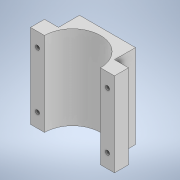
# Autodesk Inventor part: boltSideForclampForMeadeTripodLeg
Saved by Autodesk Inventor 2021.2 (Build 252289000, 289)
## iProperties
Created: 2021-02-07
Part Number: boltSideForclampForMeadeTripodLeg
Material: Generic
Document SubType Name: Modeling
Designer: robst
Density: 1 g/cm^3
Appearance: Default
Author: robst
Autodesk Inventor part; units mm, degrees
ref_plane "YZ Plane" through (0, 0, 0) normal (1, 0, 0) x (0, 1, 0)
ref_plane "XZ Plane" through (0, 0, 0) normal (0, 1, 0) x (-1, 0, 0)
ref_plane "XY Plane" through (0, 0, 0) normal (0, 0, 1) x (1, 0, 0)
sketch "Sketch18" plane through (0, 0, 0) normal (0, 1, 0) x (-1, 0, 0)
  arc A0 (-25.4, 0) -> (25.4, 0) centre (0, 0) ccw
  line L0 (-38.1, 0) -> (-38.1, -31.75)
  line L1 (-38.1, -31.75) -> (38.1, -31.75)
  line L2 (38.1, -31.75) -> (38.1, 0)
  line L3 (38.1, 31.75) -> (-38.1, -31.75) construction
  line L4 (-38.1, 31.75) -> (38.1, -31.75) construction
  line L5 (38.1, 0) -> (25.4, 0)
  line L6 (-25.4, 0) -> (-38.1, 0)
  dimension "d78" = 50.8
  dimension "d79" = 6.35
  dimension "d80" = 12.7
  constraints: 14 end point, 2 midpoint, 2 point on circle, 1 centre point, 1 coincident, 1 parallel
  measures "d78" diameter of A0
  measures "d79" distance edge to line of A0 L1
  measures "d80" distance edge to line of A0 L2
extrude "Extrusion9" add sketch "Sketch18" against normal blind 76.2
sketch "Sketch19" plane through (-38.1, 0, 0) normal (0, 0, 1) x (1, 0, 0)
  line L0 (0, 0) -> (0, -76.2) projected
  line L1 (12.7, 0) -> (12.7, -76.2) projected
  line L2 (63.5, 0) -> (63.5, -76.2) projected
  line L3 (76.2, 0) -> (76.2, -76.2) projected
  line L4 (76.2, -76.2) -> (63.5, -76.2) projected
  line L5 (12.7, -76.2) -> (0, -76.2) projected
  line L6 (0, 0) -> (12.7, 0) projected
  line L7 (63.5, 0) -> (76.2, 0) projected
  line L8 (6.35, -63.5) -> (69.85, -63.5) construction
  line L9 (69.85, -63.5) -> (69.85, -12.7) construction
  line L10 (69.85, -12.7) -> (6.35, -12.7) construction
  line L11 (6.35, -12.7) -> (6.35, -63.5) construction
  line L12 (63.5, -76.2) -> (12.7, -76.2) construction
  line L13 (12.7, 0) -> (63.5, 0) construction
  point P0 (38.1, 0)
  dimension "d83" = 6.35
  dimension "d84" = 6.35
  dimension "d85" = 12.7
  dimension "d86" = 12.7
  constraints: 8 end point, 4 coincident, 2 parallel, 1 horizontal, 1 perpendicular
  measures "d83" distance between parallel lines of L11 L0
  measures "d84" distance between parallel lines of L9 L3
  measures "d85" distance between parallel lines of L12 L8
  measures "d86" distance between parallel lines of L10 L13
hole "Hole3" at (-31.75, -12.7, 0) at (31.75, -12.7, 0) at (31.75, -63.5, 0) at (-31.75, -63.5, 0) direction (0, 0, -1) diameter 3.81 end through all clearance for "Flat Head Machine Screw (82)" size "#6" standard "Ansi Unified Screw Threads"
sketch "Sketch20" plane through (38.1, 0, -31.75) normal (0, 0, -1) x (-1, 0, 0)
  line L0 (76.2, 0) -> (76.2, -76.2) projected
  line L1 (0, 0) -> (76.2, 0) projected
  line L2 (0, 0) -> (0, -76.2) projected
  line L3 (76.2, -76.2) -> (0, -76.2) projected
  line L4 (25.4, -63.5) -> (50.8, -63.5) construction
  line L5 (50.8, -63.5) -> (50.8, -12.7) construction
  line L6 (50.8, -12.7) -> (25.4, -12.7) construction
  line L7 (25.4, -12.7) -> (25.4, -63.5) construction
  line L8 (25.4, -63.5) -> (50.8, -12.7) construction
  line L9 (50.8, -63.5) -> (25.4, -12.7) construction
  line L10 (0, 0) -> (0, -76.2) construction
  point P0 (38.1, 0)
  point P1 (38.1, -38.1)
  dimension "d94" = 12.7
  dimension "d95" = 12.7
  dimension "d96" = 25.4
  dimension "d97" = 25.4
  dimension "d110" = 25.4
  dimension "d111" = 50.8
  constraints: 12 end point, 4 coincident, 2 midpoint, 2 parallel, 2 perpendicular
  measures "d94" distance between parallel lines of L6 L1
  measures "d95" distance between parallel lines of L4 L3
  measures "d96" distance between parallel lines of L2 L7
  measures "d97" distance between parallel lines of L0 L5
  measures "d110" distance of point (25.4, -12.7) point (50.8, -12.7)
  measures "d111" distance of point (50.8, -63.5) point (50.8, -12.7)
hole "Hole4" at (12.7, -12.7, -31.75) at (-12.7, -12.7, -31.75) at (-12.7, -63.5, -31.75) at (12.7, -63.5, -31.75) direction (0, 0, 1) diameter 4.7244 depth 7.1501 counterbore diameter 5.1816 counterbore depth 5.5626
sketch "Sketch21" plane through (0, 0, 0) normal (0, 1, 0) x (1, 0, 0)
  line L0 (38.1, 31.75) -> (-38.1, 31.75) projected
  arc A0 (25.4, 0) -> (-25.4, 0) centre (0, 0) ccw projected
  line L1 (38.1, 0) -> (38.1, 31.75) projected
  line L2 (-38.1, 31.75) -> (-38.1, 0) projected
  line L3 (-38.1, 0) -> (-25.4, 0) projected
  line L4 (25.4, 0) -> (38.1, 0) projected
  line L5 (-38.1, 31.75) -> (38.1, 31.75) projected
  line L6 (-38.1, 31.75) -> (-25.4, 31.75)
  line L7 (-25.4, 31.75) -> (-25.4, 12.7)
  line L8 (-25.4, 12.7) -> (-38.1, 12.7)
  line L9 (-38.1, 12.7) -> (-38.1, 31.75)
  line L10 (38.1, 31.75) -> (25.4, 31.75)
  line L11 (25.4, 31.75) -> (25.4, 12.7)
  line L12 (25.4, 12.7) -> (38.1, 12.7)
  line L13 (38.1, 12.7) -> (38.1, 31.75)
  dimension "d105" = 19.05
  dimension "d106" = 12.7
  dimension "d107" = 19.05
  constraints: 16 end point, 4 parallel, 2 horizontal, 2 perpendicular
  measures "d105" distance of L6.end L7.end
  measures "d106" distance between parallel lines of L11 L1
  measures "d107" distance between parallel lines of L0 L12
extrude "Extrusion10" cut sketch "Sketch21" against normal through all contours L1 L12 L11 L0 | L7 L8 L2 L0
sketch "Sketch22" plane through (25.4, 0, -31.75) normal (0, 0, -1) x (-1, 0, 0)
  line L0 (0, 0) -> (0, -76.2) projected
  line L1 (0, -38.1) -> (50.8, -38.1) construction
  line L2 (50.8, 0) -> (50.8, -76.2) projected
  line L3 (19.2842, -36.576) -> (16.3103, -36.576)
  line L4 (16.3103, -36.576) -> (16.3103, -35.9536)
  line L5 (16.3103, -35.9536) -> (17.4169, -35.9536)
  line L6 (17.4169, -35.9536) -> (17.4169, -31.8681)
  line L7 (17.4169, -31.8681) -> (16.3103, -31.8681)
  line L8 (16.3103, -31.8681) -> (16.3103, -31.3099)
  spline S0 degree 2 poles (16.3103, -31.3099) (16.9377, -31.3099) (17.5305, -30.9542) (17.57, -30.4602) knots 0 0 0 1 2 2 2
  line L9 (17.57, -30.4602) -> (18.2024, -30.4602)
  line L10 (18.2024, -30.4602) -> (18.2024, -35.9536)
  line L11 (18.2024, -35.9536) -> (19.2842, -35.9536)
  line L12 (19.2842, -35.9536) -> (19.2842, -36.576)
  line L13 (21.3195, -30.2083) -> (21.1417, -32.5795)
  line L14 (21.1417, -32.5795) -> (20.6032, -32.5795)
  line L15 (20.6032, -32.5795) -> (20.4254, -30.2083)
  line L16 (20.4254, -30.2083) -> (21.3195, -30.2083)
  line L17 (22.8608, -30.2083) -> (22.683, -32.5795)
  line L18 (22.683, -32.5795) -> (22.1445, -32.5795)
  line L19 (22.1445, -32.5795) -> (21.9667, -30.2083)
  line L20 (21.9667, -30.2083) -> (22.8608, -30.2083)
  line L21 (27.4353, -36.576) -> (26.4917, -36.576)
  line L22 (26.4917, -36.576) -> (25.3802, -34.8569)
  line L23 (25.3802, -34.8569) -> (24.2391, -36.576)
  line L24 (24.2391, -36.576) -> (23.3647, -36.576)
  line L25 (23.3647, -36.576) -> (24.9505, -34.3085)
  line L26 (24.9505, -34.3085) -> (23.3795, -32.0015)
  line L27 (23.3795, -32.0015) -> (24.3231, -32.0015)
  line L28 (24.3231, -32.0015) -> (25.4296, -33.7058)
  line L29 (25.4296, -33.7058) -> (26.5609, -32.0015)
  line L30 (26.5609, -32.0015) -> (27.4353, -32.0015)
  line L31 (27.4353, -32.0015) -> (25.8594, -34.2591)
  line L32 (25.8594, -34.2591) -> (27.4353, -36.576)
  line L33 (31.6788, -36.576) -> (27.9194, -36.576)
  line L34 (27.9194, -36.576) -> (27.9194, -35.7115)
  spline S1 degree 2 poles (27.9194, -35.7115) (28.3245, -35.3311) (29.0457, -34.6247) (29.3915, -34.2443) knots 0 0 0 1 2 2 2
  spline S2 degree 2 poles (29.3915, -34.2443) (30.0881, -33.4786) (30.5969, -32.5598) (30.5969, -32.0707) knots 0 0 0 1 2 2 2
  spline S3 degree 2 poles (30.5969, -32.0707) (30.5969, -31.8138) (30.4388, -31.4285) (30.2956, -31.305) knots 0 0 0 1 2 2 2
  spline S4 degree 2 poles (30.2956, -31.305) (30.1523, -31.1815) (29.7769, -31.058) (29.5496, -31.058) knots 0 0 0 1 2 2 2
  spline S5 degree 2 poles (29.5496, -31.058) (29.3323, -31.058) (28.8877, -31.1667) (28.6851, -31.2506) knots 0 0 0 1 2 2 2
  spline S6 degree 2 poles (28.6851, -31.2506) (28.5122, -31.3198) (28.1911, -31.5174) (28.0923, -31.5866) knots 0 0 0 1 2 2 2
  line L35 (28.0923, -31.5866) -> (28.0479, -31.5866)
  line L36 (28.0479, -31.5866) -> (28.0479, -30.7171)
  spline S7 degree 2 poles (28.0479, -30.7171) (28.2998, -30.5936) (29.2038, -30.3516) (29.6089, -30.3516) knots 0 0 0 1 2 2 2
  spline S8 degree 2 poles (29.6089, -30.3516) (30.4635, -30.3516) (31.4268, -31.2556) (31.4268, -32.0262) knots 0 0 0 1 2 2 2
  spline S9 degree 2 poles (31.4268, -32.0262) (31.4268, -32.3869) (31.2589, -32.9895) (31.1107, -33.2464) knots 0 0 0 1 2 2 2
  spline S10 degree 2 poles (31.1107, -33.2464) (30.9625, -33.5132) (30.5327, -34.0368) (30.2956, -34.2888) knots 0 0 0 1 2 2 2
  spline S11 degree 2 poles (30.2956, -34.2888) (29.9102, -34.7087) (28.9667, -35.6078) (28.6851, -35.8696) knots 0 0 0 1 2 2 2
  line L37 (28.6851, -35.8696) -> (31.6788, -35.8696)
  line L38 (31.6788, -35.8696) -> (31.6788, -36.576)
  line L39 (33.4078, -30.2083) -> (33.23, -32.5795)
  line L40 (33.23, -32.5795) -> (32.6915, -32.5795)
  line L41 (32.6915, -32.5795) -> (32.5136, -30.2083)
  line L42 (32.5136, -30.2083) -> (33.4078, -30.2083)
  line L43 (34.9491, -30.2083) -> (34.7712, -32.5795)
  line L44 (34.7712, -32.5795) -> (34.2328, -32.5795)
  line L45 (34.2328, -32.5795) -> (34.0549, -30.2083)
  line L46 (34.0549, -30.2083) -> (34.9491, -30.2083)
  line L47 (7.0873, -46.7859) -> (6.3167, -46.7859)
  line L48 (6.3167, -46.7859) -> (6.3167, -44.1776)
  spline S12 degree 2 poles (6.3167, -44.1776) (6.3167, -43.8614) (6.2574, -43.318) (6.1685, -43.155) knots 0 0 0 1 2 2 2
  spline S13 degree 2 poles (6.1685, -43.155) (6.0746, -42.9821) (5.7387, -42.8142) (5.4521, -42.8142) knots 0 0 0 1 2 2 2
  spline S14 degree 2 poles (5.4521, -42.8142) (5.1656, -42.8142) (4.558, -43.1204) (4.2665, -43.3674) knots 0 0 0 1 2 2 2
  line L49 (4.2665, -43.3674) -> (4.2665, -46.7859)
  line L50 (4.2665, -46.7859) -> (3.4959, -46.7859)
  line L51 (3.4959, -46.7859) -> (3.4959, -40.4182)
  line L52 (3.4959, -40.4182) -> (4.2665, -40.4182)
  line L53 (4.2665, -40.4182) -> (4.2665, -42.7203)
  spline S15 degree 2 poles (4.2665, -42.7203) (4.6123, -42.4091) (5.2792, -42.083) (5.6547, -42.083) knots 0 0 0 1 2 2 2
  spline S16 degree 2 poles (5.6547, -42.083) (6.3265, -42.083) (7.0873, -42.9722) (7.0873, -43.817) knots 0 0 0 1 2 2 2
  line L54 (7.0873, -43.817) -> (7.0873, -46.7859)
  spline S17 degree 2 poles (11.9285, -44.4987) (11.9285, -45.6547) (10.817, -46.9144) (9.8883, -46.9144) knots 0 0 0 1 2 2 2
  spline S18 degree 2 poles (9.8883, -46.9144) (8.9349, -46.9144) (7.8431, -45.6152) (7.8431, -44.4987) knots 0 0 0 1 2 2 2
  spline S19 degree 2 poles (7.8431, -44.4987) (7.8431, -43.3526) (8.9695, -42.083) (9.8883, -42.083) knots 0 0 0 1 2 2 2
  spline S20 degree 2 poles (9.8883, -42.083) (10.817, -42.083) (11.9285, -43.3477) (11.9285, -44.4987) knots 0 0 0 1 2 2 2
  spline S21 degree 2 poles (11.1332, -44.4987) (11.1332, -43.6095) (10.486, -42.745) (9.8883, -42.745) knots 0 0 0 1 2 2 2
  spline S22 degree 2 poles (9.8883, -42.745) (9.2906, -42.745) (8.6385, -43.6095) (8.6385, -44.4987) knots 0 0 0 1 2 2 2
  spline S23 degree 2 poles (8.6385, -44.4987) (8.6385, -45.3632) (9.2906, -46.2524) (9.8883, -46.2524) knots 0 0 0 1 2 2 2
  spline S24 degree 2 poles (9.8883, -46.2524) (10.4811, -46.2524) (11.1332, -45.378) (11.1332, -44.4987) knots 0 0 0 1 2 2 2
  line L55 (13.5044, -46.7859) -> (12.7338, -46.7859)
  line L56 (12.7338, -46.7859) -> (12.7338, -40.4182)
  line L57 (12.7338, -40.4182) -> (13.5044, -40.4182)
  line L58 (13.5044, -40.4182) -> (13.5044, -46.7859)
  spline S25 degree 2 poles (16.6216, -46.8897) (15.5249, -46.8897) (14.3195, -45.6596) (14.3195, -44.5234) knots 0 0 0 1 2 2 2
  spline S26 degree 2 poles (14.3195, -44.5234) (14.3195, -43.407) (15.4903, -42.083) (16.4338, -42.083) knots 0 0 0 1 2 2 2
  spline S27 degree 2 poles (16.4338, -42.083) (16.8587, -42.083) (17.5157, -42.33) (17.7578, -42.5919) knots 0 0 0 1 2 2 2
  spline S28 degree 2 poles (17.7578, -42.5919) (18.0048, -42.8537) (18.2666, -43.6095) (18.2666, -44.1578) knots 0 0 0 1 2 2 2
  line L59 (18.2666, -44.1578) -> (18.2666, -44.5778)
  line L60 (18.2666, -44.5778) -> (15.1, -44.5778)
  spline S29 degree 2 poles (15.1, -44.5778) (15.1, -45.3731) (15.9003, -46.2178) (16.6117, -46.2178) knots 0 0 0 1 2 2 2
  spline S30 degree 2 poles (16.6117, -46.2178) (16.8636, -46.2178) (17.3527, -46.1042) (17.5503, -46.0153) knots 0 0 0 1 2 2 2
  spline S31 degree 2 poles (17.5503, -46.0153) (17.7578, -45.9165) (18.0443, -45.7436) (18.1382, -45.6646) knots 0 0 0 1 2 2 2
  line L61 (18.1382, -45.6646) -> (18.1826, -45.6646)
  line L62 (18.1826, -45.6646) -> (18.1826, -46.5044)
  spline S32 degree 2 poles (18.1826, -46.5044) (18.0492, -46.5587) (17.6441, -46.7168) (17.4861, -46.7612) knots 0 0 0 1 2 2 2
  spline S33 degree 2 poles (17.4861, -46.7612) (17.2638, -46.8255) (16.8982, -46.8897) (16.6216, -46.8897) knots 0 0 0 1 2 2 2
  spline S34 degree 2 poles (17.5157, -43.9899) (17.5058, -43.6787) (17.3774, -43.2242) (17.2539, -43.071) knots 0 0 0 1 2 2 2
  spline S35 degree 2 poles (17.2539, -43.071) (17.1205, -42.8981) (16.7006, -42.7154) (16.3894, -42.7154) knots 0 0 0 1 2 2 2
  spline S36 degree 2 poles (16.3894, -42.7154) (16.0831, -42.7154) (15.6533, -42.8981) (15.4755, -43.076) knots 0 0 0 1 2 2 2
  spline S37 degree 2 poles (15.4755, -43.076) (15.3026, -43.2588) (15.1247, -43.6984) (15.1, -43.9899) knots 0 0 0 1 2 2 2
  line L63 (15.1, -43.9899) -> (17.5157, -43.9899)
  spline S38 degree 2 poles (25.4988, -44.3752) (25.4988, -45.5213) (24.4071, -46.8749) (23.5722, -46.8749) knots 0 0 0 1 2 2 2
  spline S39 degree 2 poles (23.5722, -46.8749) (23.2313, -46.8749) (22.7077, -46.7168) (22.436, -46.5538) knots 0 0 0 1 2 2 2
  line L64 (22.436, -46.5538) -> (22.436, -48.4705)
  line L65 (22.436, -48.4705) -> (21.6653, -48.4705)
  line L66 (21.6653, -48.4705) -> (21.6653, -42.2115)
  line L67 (21.6653, -42.2115) -> (22.436, -42.2115)
  line L68 (22.436, -42.2115) -> (22.436, -42.6907)
  spline S40 degree 2 poles (22.436, -42.6907) (22.7225, -42.4288) (23.424, -42.083) (23.834, -42.083) knots 0 0 0 1 2 2 2
  spline S41 degree 2 poles (23.834, -42.083) (24.6195, -42.083) (25.4988, -43.3279) (25.4988, -44.3752) knots 0 0 0 1 2 2 2
  spline S42 degree 2 poles (24.7035, -44.4641) (24.7035, -43.6787) (24.2045, -42.8142) (23.6463, -42.8142) knots 0 0 0 1 2 2 2
  spline S43 degree 2 poles (23.6463, -42.8142) (23.3202, -42.8142) (22.7077, -43.1056) (22.436, -43.3329) knots 0 0 0 1 2 2 2
  line L69 (22.436, -43.3329) -> (22.436, -45.9313)
  spline S44 degree 2 poles (22.436, -45.9313) (22.7373, -46.0746) (23.1671, -46.1833) (23.4437, -46.1833) knots 0 0 0 1 2 2 2
  spline S45 degree 2 poles (23.4437, -46.1833) (24.0415, -46.1833) (24.7035, -45.3039) (24.7035, -44.4641) knots 0 0 0 1 2 2 2
  spline S46 degree 2 poles (28.8481, -46.3018) (28.7543, -46.371) (28.4381, -46.618) (28.2899, -46.6921) knots 0 0 0 1 2 2 2
  spline S47 degree 2 poles (28.2899, -46.6921) (28.0874, -46.8008) (27.707, -46.9144) (27.3612, -46.9144) knots 0 0 0 1 2 2 2
  spline S48 degree 2 poles (27.3612, -46.9144) (27.0796, -46.9144) (26.5708, -46.702) (26.3781, -46.5093) knots 0 0 0 1 2 2 2
  spline S49 degree 2 poles (26.3781, -46.5093) (26.1953, -46.3216) (25.973, -45.7683) (25.973, -45.462) knots 0 0 0 1 2 2 2
  spline S50 degree 2 poles (25.973, -45.462) (25.973, -44.9878) (26.3732, -44.3159) (26.8079, -44.1233) knots 0 0 0 1 2 2 2
  spline S51 degree 2 poles (26.8079, -44.1233) (27.1932, -43.9454) (28.2405, -43.812) (28.8481, -43.7775) knots 0 0 0 1 2 2 2
  line L70 (28.8481, -43.7775) -> (28.8481, -43.6293)
  spline S52 degree 2 poles (28.8481, -43.6293) (28.8481, -43.3625) (28.6851, -43.0315) (28.5369, -42.9377) knots 0 0 0 1 2 2 2
  spline S53 degree 2 poles (28.5369, -42.9377) (28.3887, -42.8438) (27.9639, -42.7845) (27.7366, -42.7845) knots 0 0 0 1 2 2 2
  spline S54 degree 2 poles (27.7366, -42.7845) (27.4699, -42.7845) (26.7486, -42.9426) (26.388, -43.0957) knots 0 0 0 1 2 2 2
  line L71 (26.388, -43.0957) -> (26.3435, -43.0957)
  line L72 (26.3435, -43.0957) -> (26.3435, -42.3103)
  spline S55 degree 2 poles (26.3435, -42.3103) (26.556, -42.251) (27.3513, -42.1028) (27.7416, -42.1028) knots 0 0 0 1 2 2 2
  spline S56 degree 2 poles (27.7416, -42.1028) (28.2158, -42.1028) (28.863, -42.251) (29.1198, -42.4437) knots 0 0 0 1 2 2 2
  spline S57 degree 2 poles (29.1198, -42.4437) (29.3718, -42.6314) (29.6188, -43.2291) (29.6188, -43.6589) knots 0 0 0 1 2 2 2
  line L73 (29.6188, -43.6589) -> (29.6188, -46.7859)
  line L74 (29.6188, -46.7859) -> (28.8481, -46.7859)
  line L75 (28.8481, -46.7859) -> (28.8481, -46.3018)
  line L76 (28.8481, -45.6596) -> (28.8481, -44.39)
  spline S58 degree 2 poles (28.8481, -44.39) (28.5715, -44.4147) (27.7366, -44.4987) (27.4748, -44.5778) knots 0 0 0 1 2 2 2
  spline S59 degree 2 poles (27.4748, -44.5778) (27.1685, -44.6716) (26.7684, -45.0619) (26.7684, -45.4077) knots 0 0 0 1 2 2 2
  spline S60 degree 2 poles (26.7684, -45.4077) (26.7684, -45.8029) (27.213, -46.203) (27.6378, -46.203) knots 0 0 0 1 2 2 2
  spline S61 degree 2 poles (27.6378, -46.203) (27.9985, -46.203) (28.5913, -45.8918) (28.8481, -45.6596) knots 0 0 0 1 2 2 2
  spline S62 degree 2 poles (32.0839, -46.8749) (31.4565, -46.8749) (30.7501, -46.1586) (30.7501, -45.383) knots 0 0 0 1 2 2 2
  line L77 (30.7501, -45.383) -> (30.7501, -42.8487)
  line L78 (30.7501, -42.8487) -> (30.2314, -42.8487)
  line L79 (30.2314, -42.8487) -> (30.2314, -42.2115)
  line L80 (30.2314, -42.2115) -> (30.7501, -42.2115)
  line L81 (30.7501, -42.2115) -> (30.7501, -40.8974)
  line L82 (30.7501, -40.8974) -> (31.5207, -40.8974)
  line L83 (31.5207, -40.8974) -> (31.5207, -42.2115)
  line L84 (31.5207, -42.2115) -> (32.9385, -42.2115)
  line L85 (32.9385, -42.2115) -> (32.9385, -42.8487)
  line L86 (32.9385, -42.8487) -> (31.5207, -42.8487)
  line L87 (31.5207, -42.8487) -> (31.5207, -45.0273)
  spline S63 degree 2 poles (31.5207, -45.0273) (31.5207, -45.3731) (31.5454, -45.7535) (31.6294, -45.9165) knots 0 0 0 1 2 2 2
  spline S64 degree 2 poles (31.6294, -45.9165) (31.6985, -46.0598) (32.0098, -46.203) (32.2765, -46.203) knots 0 0 0 1 2 2 2
  spline S65 degree 2 poles (32.2765, -46.203) (32.4642, -46.203) (32.815, -46.0894) (32.894, -46.0548) knots 0 0 0 1 2 2 2
  line L88 (32.894, -46.0548) -> (32.9385, -46.0548)
  line L89 (32.9385, -46.0548) -> (32.9385, -46.7464)
  spline S66 degree 2 poles (32.9385, -46.7464) (32.7211, -46.8057) (32.2765, -46.8749) (32.0839, -46.8749) knots 0 0 0 1 2 2 2
  spline S67 degree 2 poles (34.8898, -46.8749) (34.2624, -46.8749) (33.556, -46.1586) (33.556, -45.383) knots 0 0 0 1 2 2 2
  line L90 (33.556, -45.383) -> (33.556, -42.8487)
  line L91 (33.556, -42.8487) -> (33.0373, -42.8487)
  line L92 (33.0373, -42.8487) -> (33.0373, -42.2115)
  line L93 (33.0373, -42.2115) -> (33.556, -42.2115)
  line L94 (33.556, -42.2115) -> (33.556, -40.8974)
  line L95 (33.556, -40.8974) -> (34.3266, -40.8974)
  line L96 (34.3266, -40.8974) -> (34.3266, -42.2115)
  line L97 (34.3266, -42.2115) -> (35.7444, -42.2115)
  line L98 (35.7444, -42.2115) -> (35.7444, -42.8487)
  line L99 (35.7444, -42.8487) -> (34.3266, -42.8487)
  line L100 (34.3266, -42.8487) -> (34.3266, -45.0273)
  spline S68 degree 2 poles (34.3266, -45.0273) (34.3266, -45.3731) (34.3513, -45.7535) (34.4353, -45.9165) knots 0 0 0 1 2 2 2
  spline S69 degree 2 poles (34.4353, -45.9165) (34.5045, -46.0598) (34.8157, -46.203) (35.0825, -46.203) knots 0 0 0 1 2 2 2
  spline S70 degree 2 poles (35.0825, -46.203) (35.2702, -46.203) (35.6209, -46.0894) (35.7, -46.0548) knots 0 0 0 1 2 2 2
  line L101 (35.7, -46.0548) -> (35.7444, -46.0548)
  line L102 (35.7444, -46.0548) -> (35.7444, -46.7464)
  spline S71 degree 2 poles (35.7444, -46.7464) (35.5271, -46.8057) (35.0825, -46.8749) (34.8898, -46.8749) knots 0 0 0 1 2 2 2
  spline S72 degree 2 poles (38.2984, -46.8897) (37.2017, -46.8897) (35.9964, -45.6596) (35.9964, -44.5234) knots 0 0 0 1 2 2 2
  spline S73 degree 2 poles (35.9964, -44.5234) (35.9964, -43.407) (37.1672, -42.083) (38.1107, -42.083) knots 0 0 0 1 2 2 2
  spline S74 degree 2 poles (38.1107, -42.083) (38.5355, -42.083) (39.1926, -42.33) (39.4346, -42.5919) knots 0 0 0 1 2 2 2
  spline S75 degree 2 poles (39.4346, -42.5919) (39.6816, -42.8537) (39.9435, -43.6095) (39.9435, -44.1578) knots 0 0 0 1 2 2 2
  line L103 (39.9435, -44.1578) -> (39.9435, -44.5778)
  line L104 (39.9435, -44.5778) -> (36.7769, -44.5778)
  spline S76 degree 2 poles (36.7769, -44.5778) (36.7769, -45.3731) (37.5772, -46.2178) (38.2885, -46.2178) knots 0 0 0 1 2 2 2
  spline S77 degree 2 poles (38.2885, -46.2178) (38.5405, -46.2178) (39.0295, -46.1042) (39.2272, -46.0153) knots 0 0 0 1 2 2 2
  spline S78 degree 2 poles (39.2272, -46.0153) (39.4346, -45.9165) (39.7212, -45.7436) (39.815, -45.6646) knots 0 0 0 1 2 2 2
  line L105 (39.815, -45.6646) -> (39.8595, -45.6646)
  line L106 (39.8595, -45.6646) -> (39.8595, -46.5044)
  spline S79 degree 2 poles (39.8595, -46.5044) (39.7261, -46.5587) (39.321, -46.7168) (39.1629, -46.7612) knots 0 0 0 1 2 2 2
  spline S80 degree 2 poles (39.1629, -46.7612) (38.9406, -46.8255) (38.5751, -46.8897) (38.2984, -46.8897) knots 0 0 0 1 2 2 2
  spline S81 degree 2 poles (39.1926, -43.9899) (39.1827, -43.6787) (39.0542, -43.2242) (38.9307, -43.071) knots 0 0 0 1 2 2 2
  spline S82 degree 2 poles (38.9307, -43.071) (38.7974, -42.8981) (38.3775, -42.7154) (38.0662, -42.7154) knots 0 0 0 1 2 2 2
  spline S83 degree 2 poles (38.0662, -42.7154) (37.76, -42.7154) (37.3302, -42.8981) (37.1523, -43.076) knots 0 0 0 1 2 2 2
  spline S84 degree 2 poles (37.1523, -43.076) (36.9794, -43.2588) (36.8016, -43.6984) (36.7769, -43.9899) knots 0 0 0 1 2 2 2
  line L107 (36.7769, -43.9899) -> (39.1926, -43.9899)
  line L108 (43.1495, -43.0365) -> (43.11, -43.0365)
  spline S85 degree 2 poles (43.11, -43.0365) (43.0211, -43.0118) (42.8284, -43.0019) (42.6951, -43.0019) knots 0 0 0 1 2 2 2
  spline S86 degree 2 poles (42.6951, -43.0019) (42.3838, -43.0019) (41.7713, -43.2736) (41.4946, -43.5403) knots 0 0 0 1 2 2 2
  line L109 (41.4946, -43.5403) -> (41.4946, -46.7859)
  line L110 (41.4946, -46.7859) -> (40.724, -46.7859)
  line L111 (40.724, -46.7859) -> (40.724, -42.2115)
  line L112 (40.724, -42.2115) -> (41.4946, -42.2115)
  line L113 (41.4946, -42.2115) -> (41.4946, -42.8932)
  spline S87 degree 2 poles (41.4946, -42.8932) (41.9145, -42.5178) (42.5419, -42.2115) (42.8383, -42.2115) knots 0 0 0 1 2 2 2
  spline S88 degree 2 poles (42.8383, -42.2115) (42.9569, -42.2115) (43.0754, -42.2214) (43.1495, -42.2362) knots 0 0 0 1 2 2 2
  line L114 (43.1495, -42.2362) -> (43.1495, -43.0365)
  line L115 (47.3387, -46.7859) -> (46.568, -46.7859)
  line L116 (46.568, -46.7859) -> (46.568, -44.1776)
  spline S89 degree 2 poles (46.568, -44.1776) (46.568, -43.8614) (46.5088, -43.318) (46.4198, -43.155) knots 0 0 0 1 2 2 2
  spline S90 degree 2 poles (46.4198, -43.155) (46.326, -42.9821) (45.9901, -42.8142) (45.7035, -42.8142) knots 0 0 0 1 2 2 2
  spline S91 degree 2 poles (45.7035, -42.8142) (45.417, -42.8142) (44.8094, -43.1204) (44.5179, -43.3674) knots 0 0 0 1 2 2 2
  line L117 (44.5179, -43.3674) -> (44.5179, -46.7859)
  line L118 (44.5179, -46.7859) -> (43.7473, -46.7859)
  line L119 (43.7473, -46.7859) -> (43.7473, -42.2115)
  line L120 (43.7473, -42.2115) -> (44.5179, -42.2115)
  line L121 (44.5179, -42.2115) -> (44.5179, -42.7203)
  spline S92 degree 2 poles (44.5179, -42.7203) (44.8637, -42.4091) (45.5306, -42.083) (45.9061, -42.083) knots 0 0 0 1 2 2 2
  spline S93 degree 2 poles (45.9061, -42.083) (46.5779, -42.083) (47.3387, -42.9722) (47.3387, -43.817) knots 0 0 0 1 2 2 2
  line L122 (47.3387, -43.817) -> (47.3387, -46.7859)
  point P0 (25.4, 0)
  constraints: 2 end point, 2 midpoint, 1 horizontal
extrude "Extrusion11" cut sketch "Sketch22" against normal blind 1.27
equation "\"d78\" = legDiameter"
equation "\"d81\" = legPartHeight"
equation "\"d98\" = diameterOfBottomOfHeatInsert"
equation "\"d100\" = diameterOfTopOfHeatInsert"
equation "\"d101\" = heightOfTopOfHeatInsert"
equation "\"d103\" = heightOfBottomOfHeatInsert"
equation "\"legDiameter\" = 50.8"
equation "\"legWalThickness\" = 3.175"
equation "\"legPartHeight\" = 76.2"
equation "\"heightOfBottomOfHeatInsert\" = 1.5875"
equation "\"heightOfTopOfHeatInsert\" = 5.5626"
equation "\"diameterOfBottomOfHeatInsert\" = 4.7244"
equation "\"diameterOfTopOfHeatInsert\" = 5.1816"
body "Solid1"
body "Solid2"
